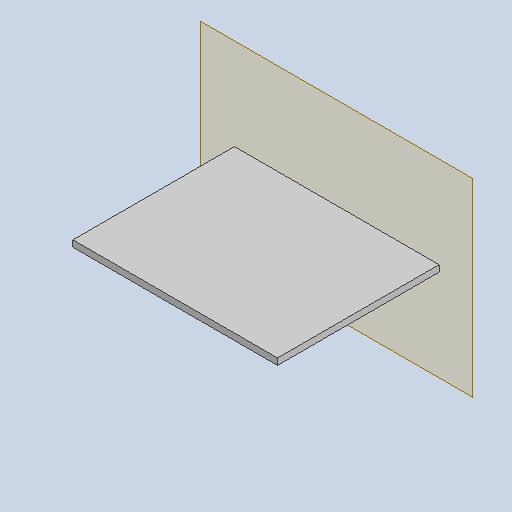
# Autodesk Inventor part: Деталь2
Saved by Autodesk Inventor 2023.1 (Build 271208000, 208)
## iProperties
Created: 2024-11-19
Part Number: Деталь2
Material: Типовые
Document SubType Name: Modeling
Designer: DELL
Density: 1 g/cm^3
Appearance: По умолчанию
Author: DELL
Autodesk Inventor part; units mm, degrees
ref_plane "YZ Plane" through (0, 0, 0) normal (1, 0, 0) x (0, 1, 0)
ref_plane "XZ Plane" through (0, 0, 0) normal (0, 1, 0) x (-1, 0, 0)
ref_plane "XY Plane" through (0, 0, 0) normal (0, 0, 1) x (1, 0, 0)
ref_plane "РабПлоскость1" through (0, 0, 50) normal (0, 0, 1) x (1, 0, 0)
sketch "Эскиз1" plane through (0, 0, 50) normal (0, 0, 1) x (1, 0, 0)
  ellipse E0 centre (0, 0) end of major axis (-114.9977, 0.7305) minor radius 79.9992 projected
  line L0 (95, 3) -> (-95, 3)
  line L1 (-95, 3) -> (-95, -3)
  line L2 (-95, -3) -> (95, -3)
  line L3 (95, -3) -> (95, 3)
  line L4 (95, 3) -> (-95, -3) construction
  line L5 (-95, 3) -> (95, -3) construction
  point P0 (0, 0)
  dimension "d0" = 190
  dimension "d1" = 6
  constraints: 12 end point, 2 midpoint, 2 parallel, 1 horizontal, 1 perpendicular, 1 other
  measures "d0" distance of L2.end L1.end
  measures "d1" distance of L1.end L0.end
extrude "Выдавливание1" add sketch "Эскиз1" along normal blind 150 contours L3 L2 L1 L0
